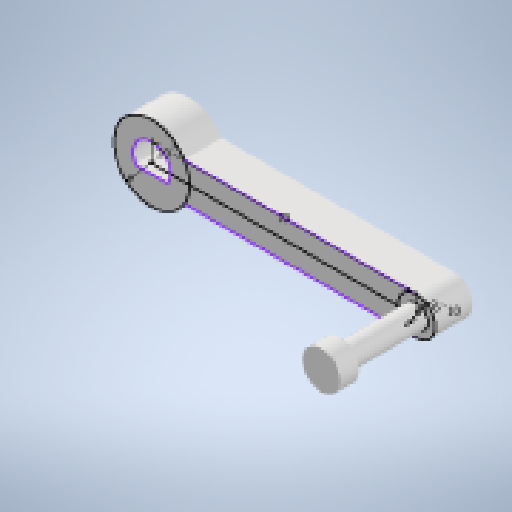
# Autodesk Inventor part: Cranker1
Saved by Autodesk Inventor 2024 (Build 280153000, 153)
## iProperties
Created: 2024-10-17
Part Number: Cranker1
Material: 一般
Document SubType Name: Modeling
Designer: jerry
Density: 1 g/cm^3
Appearance: 預設
Author: jerry
Autodesk Inventor part; units mm, degrees
ref_plane "YZ Plane" through (0, 0, 0) normal (1, 0, 0) x (0, 1, 0)
ref_plane "XZ Plane" through (0, 0, 0) normal (0, 1, 0) x (-1, 0, 0)
ref_plane "XY Plane" through (0, 0, 0) normal (0, 0, 1) x (1, 0, 0)
sketch "草圖2" plane through (0, 0, 0) normal (0, 0, 1) x (1, 0, 0)
  line L0 (4.3301, -2.5) -> (-4.3301, -2.5)
  arc A0 (4.3301, -2.5) -> (-4.3301, -2.5) centre (0, 0) ccw
  circle A1 centre (0, 0) radius 10
  line L1 (0, 0) -> (70, 0)
  circle A2 centre (70, 0) radius 5
  line L2 (8.6603, 5) -> (70, 5)
  line L3 (70, -5) -> (8.6603, -5)
  circle A3 centre (70, 0) radius 3
  dimension "d2" = 20
  dimension "d3" = 70
  dimension "d4" = 10
  dimension "d7" = 6
  constraints: 8 end point, 6 point on circle, 4 centre point, 4 coincident, 2 tangent, 1 horizontal, 1 parallel
  measures "d2" diameter of A1
  measures "d3" distance of L1.start L1.end
  measures "d4" diameter of A2
  measures "d7" diameter of A3
extrude "擠出1" add sketch "草圖2" against normal blind 10 contours A1 | A1 L2 A2 L1 | L1 A2 L3 A1 | A3 | A2
extrude "擠出2" add sketch "草圖2" along normal blind 20 contours A3
sketch "草圖3" plane through (70, 0, 20) normal (0, 0, 1) x (1, 0, 0)
  circle A0 centre (0, 0) radius 5
  point P0 (-70, 0)
  dimension "d10" = 10
  constraints: 1 centre point
  measures "d10" diameter of A0
extrude "擠出3" add sketch "草圖3" along normal blind 5
